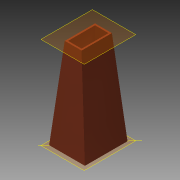
# Autodesk Inventor part: NewHorn
Saved by Autodesk Inventor 2015 (Build 190159000, 159)
## iProperties
Created: 2014-03-24
Part Number: NewHorn
Material: Copper
Document SubType Name: Modeling
Designer: jad211
Density: 8.94 g/cm^3
Appearance: Copper - Satin
Author: jad211
Autodesk Inventor part; units mm, degrees
ref_plane "YZ Plane" through (0, 0, 0) normal (1, 0, 0) x (0, 1, 0)
ref_plane "XZ Plane" through (0, 0, 0) normal (0, 1, 0) x (-1, 0, 0)
ref_plane "XY Plane" through (0, 0, 0) normal (0, 0, 1) x (1, 0, 0)
sketch "Sketch1" plane through (0, 0, 0) normal (0, 0, 1) x (1, 0, 0)
  line L0 (-10.5, -12.5) -> (10.5, -12.5)
  line L1 (10.5, -12.5) -> (10.5, 12.5)
  line L2 (10.5, 12.5) -> (-10.5, 12.5)
  line L3 (-10.5, 12.5) -> (-10.5, -12.5)
  line L4 (-10.5, -12.5) -> (10.5, 12.5) construction
  line L5 (10.5, -12.5) -> (-10.5, 12.5) construction
  point P0 (0, 0)
  dimension "d0" = 21
  dimension "d1" = 25
  constraints: 12 end point, 2 midpoint, 2 parallel, 1 horizontal, 1 perpendicular
  measures "d0" distance of L2.end L1.end
  measures "d1" distance of L1.end L0.end
ref_plane "Work Plane2" through (10.5, -12.5, 54) normal (0, 0, 1) x (0, 1, 0)
ref_plane "Work Plane1" through (10.5, -12.5, 0) normal (0, 0, 1) x (0, 1, 0)
sketch "Sketch2" plane through (10.5, -12.5, 54) normal (0, 0, 1) x (0, 1, 0)
  line L0 (3.6005, 5.5505) -> (21.3995, 5.5505)
  line L1 (21.3995, 5.5505) -> (21.3995, 15.4495)
  line L2 (21.3995, 15.4495) -> (3.6005, 15.4495)
  line L3 (3.6005, 15.4495) -> (3.6005, 5.5505)
  line L4 (3.6005, 5.5505) -> (21.3995, 15.4495) construction
  line L5 (21.3995, 5.5505) -> (3.6005, 15.4495) construction
  point P0 (12.5, 10.5)
  dimension "d3" = 17.799
  dimension "d4" = 9.899
  constraints: 12 end point, 2 midpoint, 2 parallel, 1 horizontal, 1 perpendicular
  measures "d3" distance of L2.end L1.end
  measures "d4" distance of L1.end L0.end
loft "Loft1" add profiles "Sketch2", "Sketch1"
sketch "Sketch4" plane through (10.5, -12.5, 0) normal (0, 0, -1) x (-1, 0, 0)
  line L0 (1, 1) -> (20, 1)
  line L1 (20, 1) -> (20, 24)
  line L2 (20, 24) -> (1, 24)
  line L3 (1, 24) -> (1, 1)
  line L4 (1, 1) -> (20, 24) construction
  line L5 (20, 1) -> (1, 24) construction
  point P0 (10.5, 12.5)
  dimension "d9" = 19
  dimension "d10" = 23
  constraints: 12 end point, 2 midpoint, 2 parallel, 1 horizontal, 1 perpendicular
  measures "d9" distance of L2.end L1.end
  measures "d10" distance of L1.end L0.end
sketch "Sketch5" plane through (-4.9495, 8.8995, 54) normal (0, 0, 1) x (1, 0, 0)
  line L0 (1, -16.799) -> (8.899, -16.799)
  line L1 (8.899, -16.799) -> (8.899, -1)
  line L2 (8.899, -1) -> (1, -1)
  line L3 (1, -1) -> (1, -16.799)
  line L4 (1, -16.799) -> (8.899, -1) construction
  line L5 (8.899, -16.799) -> (1, -1) construction
  point P0 (4.9495, -8.8995)
  dimension "d11" = 7.899
  dimension "d12" = 15.799
  constraints: 12 end point, 2 midpoint, 2 parallel, 1 horizontal, 1 perpendicular
  measures "d11" distance of L2.end L1.end
  measures "d12" distance of L1.end L0.end
loft "Loft2" cut profiles "Sketch5", "Sketch4"
body "Solid1"
